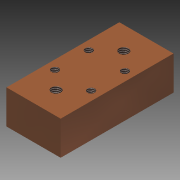
# Autodesk Inventor part: 13_0204_029
Saved by Autodesk Inventor 2012 SP1 (Build 160190100, 190)
## iProperties
Created: 2013-04-05
Part Number: 13_0204_029
Material: Default
Document SubType Name: Modeling
Designer: vogel
Density: 1 g/cm^3
Author: vogel
Autodesk Inventor part; units mm, degrees
ref_plane "YZ Plane" through (0, 0, 0) normal (1, 0, 0) x (0, 1, 0)
ref_plane "XZ Plane" through (0, 0, 0) normal (0, 1, 0) x (-1, 0, 0)
ref_plane "XY Plane" through (0, 0, 0) normal (0, 0, 1) x (1, 0, 0)
sketch "Skizze1" plane through (0, 0, 0) normal (0, 0, 1) x (1, 0, 0)
  line L0 (-12, 25) -> (12, 25)
  line L1 (12, 25) -> (12, -25)
  line L2 (12, -25) -> (-12, -25)
  line L3 (-12, -25) -> (-12, 25)
  line L4 (-16.8, 0) -> (16.8, 0) projected
  line L5 (0, -35) -> (0, 35) projected
  point P0 (0, 0)
  dimension "d0" = 24
  dimension "d1" = 50
  constraints: 8 end point, 2 parallel, 1 horizontal, 1 perpendicular, 2 other
  measures "d0" distance of L0.start L0.end
  measures "d1" distance of L2.end L0.start
extrude "Extrusion1" add sketch "Skizze1" along normal blind 15
sketch "Skizze2" plane through (0, 0, 15) normal (0, 0, 1) x (1, 0, 0)
  line L0 (-16.8, 0) -> (16.8, 0) projected
  line L1 (0, -35) -> (0, 35) projected
  line L2 (-8, 7.5) -> (8, 7.5)
  line L3 (8, 7.5) -> (8, -7.5)
  line L4 (8, -7.5) -> (-8, -7.5)
  line L5 (-8, -7.5) -> (-8, 7.5)
  point P0 (0, 0)
  dimension "d4" = 16
  dimension "d5" = 15
  constraints: 8 end point, 4 coincident, 2 parallel, 1 horizontal, 1 perpendicular, 2 other
  measures "d4" distance of L2.start L2.end
  measures "d5" distance of L2.end L3.end
hole "Bohrung1" at (-8, 7.5, 15) at (8, 7.5, 15) at (8, -7.5, 15) at (-8, -7.5, 15) direction (0, 0, -1) diameter 3.242 end through all thread size "M4x0.7" class "6H" standard "ISO Metric profile"
sketch "Skizze3" plane through (0, 0, 15) normal (0, 0, 1) x (1, 0, 0)
  circle A0 centre (0, 15) radius 2.75 projected
  circle A1 centre (0, -15) radius 2.75 projected
  point P0 (0, 0)
  constraints: 2 coincident
hole "Bohrung2" at (0, 15, 15) at (0, -15, 15) direction (0, 0, -1) diameter 4.134 end through all thread size "M5x0.8" class "6H" standard "ISO Metric profile"
